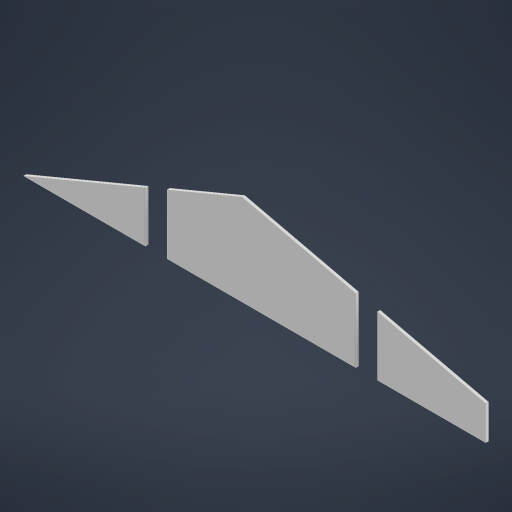
# Autodesk Inventor part: Langbektang houder
Saved by Autodesk Inventor 2023.2 (Build 272271000, 271)
## iProperties
Created: 2020-09-09
Part Number: Langbektang houder
Material: Generic
Document SubType Name: Modeling
Designer: nathan.bollaert
Density: 1 g/cm^3
Appearance: Default
Author: nathan.bollaert
Autodesk Inventor part; units mm, degrees
ref_plane "YZ Plane" through (0, 0, 0) normal (1, 0, 0) x (0, 1, 0)
ref_plane "XZ Plane" through (0, 0, 0) normal (0, 1, 0) x (-1, 0, 0)
ref_plane "XY Plane" through (0, 0, 0) normal (0, 0, 1) x (1, 0, 0)
sketch "Sketch1" plane through (0, 0, 0) normal (0, 0, 1) x (1, 0, 0)
  line L0 (13.8455, -58.3807) -> (313.7199, -67.0622)
  line L1 (313.7199, -67.0622) -> (333.7863, 0)
  line L2 (13.8455, -58.3807) -> (0, 0)
  line L3 (0, 0) -> (333.7863, 0)
  line L4 (120, 50) -> (333.7863, 0)
  line L5 (120, 50) -> (0, 0)
  line L6 (120.6929, 41.6221) -> (40, 8)
  line L7 (210.6929, 8) -> (210.6929, 20.573)
  line L8 (210.6929, 20.573) -> (120.6929, 41.6221)
  line L9 (85, 26.75) -> (85, 8)
  line L10 (120.6929, 41.6221) -> (122.5148, 49.4118)
  line L11 (120.6929, 41.6221) -> (117.616, 49.0067)
  line L12 (210.6929, 8) -> (210.6929, 0)
  line L13 (170.6929, 29.9281) -> (170.6929, 8)
  line L14 (93, 30.0833) -> (93, 8)
  line L15 (85, 8) -> (93, 8)
  line L16 (162.6929, 31.7992) -> (162.6929, 8)
  line L17 (162.6929, 8) -> (170.6929, 8)
  line L18 (210.6929, 8) -> (40, 8)
  point P0 (170.6929, 8)
  dimension "d228" = 105
  dimension "d268" = 60
  dimension "d269" = 70
  dimension "d270" = 300
  dimension "d273" = 120
  dimension "d274" = 50
  dimension "d275" = 105
  dimension "d283" = 90
  dimension "d284" = 40
  dimension "d285" = 45
  dimension "d289" = 8
  dimension "d290" = 8
  constraints: 38 end point, 10 point on line, 3 equal length, 3 horizontal, 3 parallel, 3 perpendicular, 3 vertical, 1 coincident
  measures "d228" angle of L1 L0
  measures "d268" distance of L0.start L3.start
  measures "d269" distance of L0.end L3.end
  measures "d270" distance of L0.start L0.end
  measures "d273" horizontal distance of point (0, 0) L4.start
  measures "d274" vertical distance of point (0, 0) L4.start
  measures "d275" angle of L0 L2
  measures "d283" horizontal distance of L6.start L7.end
  measures "d284" horizontal distance of L7.end L13.start
  measures "d285" horizontal distance of L6.end L9.start
  measures "d289" distance between parallel lines of L9 L14
  measures "d290" distance from line of L3 L6.end
extrude "Extrusion1" add sketch "Sketch1" against normal blind 2.5 contours L18 L13 L8 L7 | L8 L16 L18 L14 L6 | L9 L18 L6
extrude "Extrusion2" cut sketch "Sketch1" against normal blind 1.5 contours L18 L13 L8 L7 | L8 L16 L18 L14 L6 | L9 L18 L6
body "Solid5"
